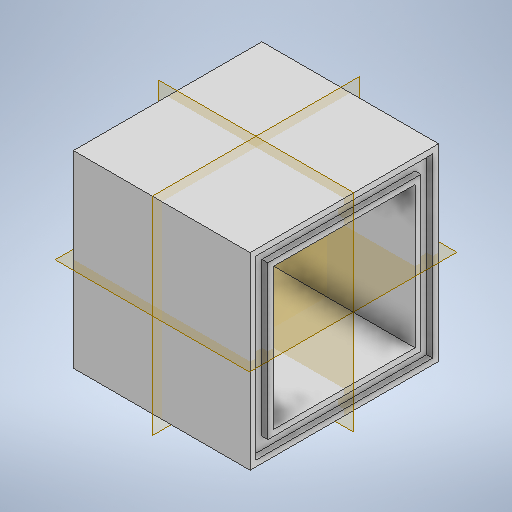
# Autodesk Inventor part: peca_010_001
Saved by Autodesk Inventor 2026 (Build 300175000, 175)
## iProperties
Created: 2025-03-26
Part Number: peca_010_001
Material: Generic
Document SubType Name: Modeling
Designer: Carlos Dias
Density: 1 g/cm^3
Appearance: Default
Author: Carlos Dias
Autodesk Inventor part; units mm, degrees
sketch "Sketch1" plane through (0, 0, 0) normal (1, 0, 0) x (0, 1, 0)
  line L0 (8, 8) -> (-8, 8)
  line L1 (-8, 8) -> (-8, -8)
  line L2 (-8, -8) -> (8, -8)
  line L3 (8, -8) -> (8, 8)
  line L4 (8, 8) -> (-8, -8) construction
  line L5 (-8, 8) -> (8, -8) construction
  line L6 (6, 6) -> (-6, 6)
  line L7 (-6, 6) -> (-6, -6)
  line L8 (-6, -6) -> (6, -6)
  line L9 (6, -6) -> (6, 6)
  line L10 (6, 6) -> (-6, -6) construction
  line L11 (-6, 6) -> (6, -6) construction
  point P0 (0, 0)
  point P1 (0, 0)
  dimension "d0" = 6
  dimension "d1" = 2
  constraints: 24 end point, 4 midpoint, 4 parallel, 3 perpendicular, 2 coincident, 2 horizontal, 1 point on line
  measures "d0" distance from line of point (0, 0) L9
  measures "d1" distance between parallel lines of L9 L3
extrude "Extrusion1" add sketch "Sketch1" along normal mid plane 15
sketch "Sketch2" plane through (7.5, 0, 0) normal (1, 0, 0) x (0, 0, -1)
  line L0 (7, 7) -> (-7, 7)
  line L1 (-7, 7) -> (-7, -7)
  line L2 (-7, -7) -> (7, -7)
  line L3 (7, -7) -> (7, 7)
  point P0 (0, 0)
  point P1 (0, 7)
  point P2 (7, 0)
  dimension "d4" = 14
  dimension "d5" = 14
  constraints: 9 end point, 2 midpoint, 1 horizontal, 1 horizontal alignment, 1 parallel, 1 perpendicular, 1 vertical, 1 vertical alignment
  measures "d4" distance of L0.start L0.end
  measures "d5" distance between parallel lines of L2 L0
sketch "Sketch3" plane through (0, 0, 0) normal (0, 1, 0) x (-1, 0, 0)
  line L0 (-8, 6.5) -> (-7, 6.5)
  line L1 (-7, 6.5) -> (-7, 7.5)
  line L2 (-7, 7.5) -> (-8, 7.5)
  line L3 (-8, 7.5) -> (-8, 6.5)
  line L4 (-8, 6.5) -> (-7, 7.5) construction
  line L5 (-7, 6.5) -> (-8, 7.5) construction
  line L6 (-7.5, 8) -> (-7.5, -8) projected
  point P0 (0, 0)
  point P1 (-7.5, 7)
  point P2 (-7.5, 0)
  dimension "d6" = 1
  dimension "d7" = 7
  constraints: 12 end point, 3 midpoint, 2 parallel, 2 perpendicular, 1 horizontal, 1 point on line
  measures "d6" distance of L2.end L0.start
  measures "d7" distance of point (-7.5, 0) point (-7.5, 7)
sweep "Sweep1" cut profiles "Sketch3" path "Sketch2" path curves L3 L2 L1 L0
sketch "Sketch4" plane through (0, 0, 0) normal (1, 0, 0) x (0, 1, 0)
  point P0 (0, 0)
sketch "Sketch5" plane through (0, 0, 0) normal (0, 1, 0) x (-1, 0, 0)
  point P0 (0, 0)
body "Solid1"
